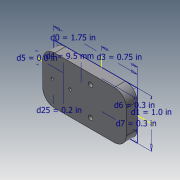
# Autodesk Inventor part: VP TRAY SWITCH MOUNT
Saved by Autodesk Inventor 2018.3 (Build 223284000, 284)
## iProperties
Created: 2020-01-28
Material: Generic
Vendor: HHMI: JRC - ID&F
Document SubType Name: Modeling
Designer: arnoldj
Density: 1 g/cm^3
Appearance: Default
RuleStatus: InUse
AfterDocSave0: file://Part Number Cleaner
DESIGN DEPARTMENT: HHMI: JRC - ID&F
ALTERED ITEM PART NUMBER: N/A
ALTERED ITEM VENDOR: N/A
ALTERED ITEM DESCRIPTION: N/A
Author: arnoldj
Revision Number: 0
Autodesk Inventor part; units mm, degrees
ref_plane "YZ Plane" through (0, 0, 0) normal (1, 0, 0) x (0, 1, 0)
ref_plane "XZ Plane" through (0, 0, 0) normal (0, 1, 0) x (-1, 0, 0)
ref_plane "XY Plane" through (0, 0, 0) normal (0, 0, 1) x (1, 0, 0)
sketch "Sketch1" plane through (0, 0, 0) normal (0, 0, 1) x (1, 0, 0)
  line L0 (0, 17.78) -> (0, -17.78) projected
  line L1 (-34.29, 0) -> (27.94, 0) projected
  line L2 (-25.4, -12.7) -> (19.05, -12.7)
  line L3 (19.05, -12.7) -> (19.05, 12.7)
  line L4 (19.05, 12.7) -> (-25.4, 12.7)
  line L5 (-25.4, 12.7) -> (-25.4, -12.7)
  line L6 (-25.4, -12.7) -> (19.05, 12.7) construction
  line L7 (19.05, -12.7) -> (-25.4, 12.7) construction
  line L8 (-20.32, 0) -> (-10.82, 0) construction
  point P0 (0, 0)
  point P1 (-3.175, 0)
  point P2 (-15.57, 0)
  point P3 (0, 7.62)
  point P4 (0, -7.62)
  dimension "d0" = 44.45
  dimension "d1" = 25.4
  dimension "d3" = 19.05
  dimension "d4" = 9.5
  dimension "d5" = 0
  dimension "d6" = 7.62
  dimension "d7" = 7.62
  dimension "d25" = 5.08
  constraints: 14 end point, 4 midpoint, 2 coincident, 2 horizontal, 2 parallel, 2 point on line, 1 perpendicular
  measures "d0" distance of L3.end L4.end
  measures "d1" distance of L2.end L3.end
  measures "d3" distance between parallel lines of L3 L0
  measures "d4" distance of L8.start L8.end
  measures "d5" distance between parallel lines of L8 L1
  measures "d6" distance from line of L1 point (0, 7.62)
  measures "d7" distance from line of L1 point (0, -7.62)
  measures "d25" distance from line of L5 point (-20.32, 0)
extrude "Extrusion1" add sketch "Sketch1" along normal blind 5.842
hole "Hole1" at (-20.32, 0, 0) at (-10.82, 0, 0) direction (0, 0, 1) diameter 1.4986 end through all
hole "Hole2" at (0, 7.62, 0) at (0, -7.62, 0) direction (0, 0, 1) diameter 2.3622 end through all
fillet "Fillet1" radius 6.35 4 edges at (19.05, 12.7, 2.921) (-25.4, 12.7, 2.921) (-25.4, -12.7, 2.921) (19.05, -12.7, 2.921)
body "Solid1"
